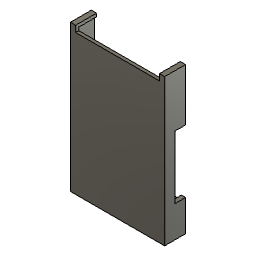
Case (Autodesk Fusion 360 archive; units mm, degrees)
design "Back Plate"
Autodesk Fusion 360 part; units mm, degrees
sketch "Sketch1" plane through (0, 0, 0) normal (0, 1, 0) x (1, 0, 0)
  line L0 (0, 0) -> (90, 0)
  line L1 (90, 0) -> (90, 20)
  line L2 (90, 20) -> (0, 20)
  line L3 (0, 20) -> (0, 0)
  dimension "d1" = 90
  dimension "d2" = 20
  constraint horizontal L0
  constraint vertical L1
  constraint horizontal L2
  constraint vertical L3
  constraint coincident L0.start L3.end
  measures "d1" distance of L0.start L0.end
  measures "d2" distance of L0.start L2.end
extrude "Extrude1" add sketch "Sketch1" along normal blind 140
shell "Shell1" thickness 3 removed faces 1 at (60, 46.6667, -20)
sketch "Sketch2" plane through (0, 0, -20) normal (0, 0, -1) x (-1, 0, 0)
  line L0 (-3, 137) -> (-3, 3)
  line L1 (-3, 3) -> (-87, 3)
  line L2 (-87, 3) -> (-87, 137)
  line L3 (-87, 137) -> (-3, 137)
  line L4 (-90, 0) -> (0, 0)
  line L5 (0, 0) -> (0, 140)
  line L6 (0, 140) -> (-90, 140)
  line L7 (-90, 140) -> (-90, 0)
  line L8 (-87, 30) -> (-90, 30)
  line L9 (-90, 30) -> (-90, 90)
  line L10 (-90, 90) -> (-87, 90)
  line L11 (-87, 90) -> (-87, 30)
  line L12 (0, 3) -> (-3, 3)
  line L13 (-3, 3) -> (-3, 18)
  line L14 (-3, 18) -> (0, 18)
  line L15 (0, 18) -> (0, 3)
  dimension "d6" = 60
  dimension "d9" = 30
  dimension "d10" = 15
  constraint horizontal L8
  constraint vertical L9
  constraint horizontal L10
  constraint vertical L11
  constraint coincident L7 L9.end
  constraint coincident L2 L8.start
  constraint horizontal L12
  constraint vertical L13
  constraint horizontal L14
  constraint vertical L15
  constraint coincident L5 L12.start
  measures "d6" distance of L8.start L10.end
  measures "d9" distance of L4 L8
  measures "d10" distance of L12.start L14.end
extrude "Extrude2" cut sketch "Sketch2" against normal blind 10 contours L2 L7 L8 L9 L10 L11
extrude "Extrude3" cut sketch "Sketch2" against normal blind 10 contours L0 L5 L12 L13 L14 L15
sketch "Sketch3" plane through (0, 0, -3) normal (0, 0, -1) x (-1, 0, 0)
  line L0 (-87, 3) -> (-3, 3)
  line L1 (-3, 3) -> (-3, 137)
  line L2 (-3, 137) -> (-87, 137)
  line L3 (-87, 137) -> (-87, 3)
  line L4 (-87, 30) -> (-80, 30)
  line L5 (-80, 30) -> (-80, 25)
  line L6 (-80, 25) -> (-87, 25)
  line L7 (-87, 25) -> (-87, 30)
  line L8 (-35, 30) -> (-28, 30)
  line L9 (-28, 30) -> (-28, 25)
  line L10 (-28, 25) -> (-35, 25)
  line L11 (-35, 25) -> (-35, 30)
  dimension "d13" = 45
  constraint horizontal L4
  constraint vertical L5
  constraint horizontal L6
  constraint vertical L7
  constraint coincident L3 L4.start
  constraint horizontal L8
  constraint vertical L9
  constraint horizontal L10
  constraint vertical L11
  measures "d13" distance of L5 L11
extrude "Extrude4" add sketch "Sketch3" along normal blind 17 contours L3 L4 L5 L6 L7 | L8 L9 L10 L11
sketch "Sketch4" plane through (0, 0, -20) normal (0, 0, -1) x (-1, 0, 0)
  line L0 (-35, 25) -> (-28, 25)
  line L1 (-28, 25) -> (-28, 30)
  line L2 (-28, 30) -> (-35, 30)
  line L3 (-35, 30) -> (-35, 25)
  line L4 (-35, 30.6629) -> (-29, 30.6629)
  line L5 (-29, 30.6629) -> (-29, 26)
  line L6 (-29, 26) -> (-35, 26)
  line L7 (-35, 26) -> (-35, 30.6629)
  constraint horizontal L4
  constraint vertical L5
  constraint horizontal L6
  constraint vertical L7
  constraint coincident L3 L4.start
sketch "Sketch5" plane through (0, 0, -20) normal (0, 0, -1) x (-1, 0, 0)
  line L0 (0, 3) -> (-87, 3)
  line L1 (-87, 3) -> (-87, 25)
  line L2 (-87, 25) -> (-80, 25)
  line L3 (-80, 25) -> (-80, 30)
  line L4 (-80, 30) -> (-90, 30)
  line L5 (-90, 30) -> (-90, 0)
  line L6 (-90, 0) -> (0, 0)
  line L7 (0, 0) -> (0, 3)
  line L8 (-80, 30) -> (-86, 30)
  line L9 (-86, 30) -> (-86, 26)
  line L10 (-86, 26) -> (-80, 26)
  line L11 (-80, 26) -> (-80, 30)
  constraint horizontal L8
  constraint vertical L9
  constraint horizontal L10
  constraint vertical L11
  constraint coincident L3.end L4.start
extrude "Extrude5" cut sketch "Sketch5" sketch "Sketch4" against normal blind 17 contours L3 L4 L8 L9 L10 L11 of sketch 2 contours L2 L4 L5 L7
extrude "Extrude6" cut sketch "Sketch4" against normal blind 17 contours L2 L3 L5 L6 L7
sketch "Sketch6" plane through (0, 0, -3) normal (0, 0, -1) x (-1, 0, 0)
  line L0 (-29, 30) -> (-28, 30)
  line L1 (-28, 30) -> (-28, 25)
  line L2 (-28, 25) -> (-35, 25)
  line L3 (-35, 25) -> (-35, 26)
  line L4 (-35, 26) -> (-29, 26)
  line L5 (-29, 26) -> (-29, 30)
  line L6 (-87, 30) -> (-86, 30)
  line L7 (-86, 30) -> (-86, 26)
  line L8 (-86, 26) -> (-80, 26)
  line L9 (-80, 26) -> (-80, 25)
  line L10 (-80, 25) -> (-87, 25)
  line L11 (-87, 25) -> (-87, 3)
  line L12 (-87, 3) -> (-3, 3)
  line L13 (-3, 3) -> (-3, 137)
  line L14 (-3, 137) -> (-87, 137)
  line L15 (-87, 137) -> (-87, 30)
  line L16 (-43, 3) -> (-48, 3)
  line L17 (-48, 3) -> (-48, 7)
  line L18 (-48, 7) -> (-43, 7)
  line L19 (-43, 7) -> (-43, 3)
  line L20 (-43, 7) -> (-47, 7)
  line L21 (-47, 7) -> (-47, 3)
  line L22 (-47, 3) -> (-43, 3)
  line L23 (-43, 3) -> (-43, 7)
  dimension "d20" = 40
  constraint horizontal L16
  constraint vertical L17
  constraint horizontal L18
  constraint vertical L19
  constraint coincident L12 L16.start
  constraint horizontal L20
  constraint vertical L21
  constraint horizontal L22
  constraint vertical L23
  constraint coincident L12 L21.end
  measures "d20" distance of L13 L19
extrude "Extrude7" add sketch "Sketch6" along normal blind 17 contours L12 L16 L17 L18 L21
sketch "Sketch7" plane through (0, 0, -3) normal (0, 0, -1) x (-1, 0, 0)
  line L0 (-48, 3) -> (-48, 7)
  line L1 (-48, 7) -> (-47, 7)
  line L2 (-47, 7) -> (-47, 3)
  line L3 (-47, 3) -> (-3, 3)
  line L4 (-3, 3) -> (-3, 137)
  line L5 (-3, 137) -> (-87, 137)
  line L6 (-87, 137) -> (-87, 30)
  line L7 (-87, 30) -> (-86, 30)
  line L8 (-86, 30) -> (-86, 26)
  line L9 (-86, 26) -> (-80, 26)
  line L10 (-80, 26) -> (-80, 25)
  line L11 (-80, 25) -> (-87, 25)
  line L12 (-87, 25) -> (-87, 3)
  line L13 (-87, 3) -> (-48, 3)
  line L14 (-29, 30) -> (-28, 30)
  line L15 (-28, 30) -> (-28, 25)
  line L16 (-28, 25) -> (-35, 25)
  line L17 (-35, 25) -> (-35, 26)
  line L18 (-35, 26) -> (-29, 26)
  line L19 (-29, 26) -> (-29, 30)
  line L20 (-47, 3) -> (-3, 3)
  line L21 (-3, 3) -> (-3, 18)
  line L22 (-3, 18) -> (-47, 18)
  line L23 (-47, 18) -> (-47, 3)
  constraint horizontal L20
  constraint vertical L21
  constraint horizontal L22
  constraint vertical L23
  constraint coincident L4 L21.end
  constraint coincident L2.end L3.start
extrude "Extrude8" add sketch "Sketch7" along normal blind 7 contours L2 L3 L4 L20 L21 L22 L23
extrude "Extrude9" add 1 faces at (47.6667, 7, -11) along direction (0, 1, 0) blind 11
sketch "Sketch8" plane through (0, 140, 0) normal (0, 1, 0) x (-1, 0, 0)
  line L0 (0, -20) -> (0, 0)
  line L1 (0, 0) -> (-90, 0)
  line L2 (-90, 0) -> (-90, -20)
  line L3 (-90, -20) -> (0, -20)
  line L4 (-90, -8) -> (-85, -8) construction
  line L5 (-85, -20) -> (-5, -20)
  line L6 (-5, -20) -> (-5, 0)
  line L7 (-5, 0) -> (-85, 0)
  line L8 (-85, 0) -> (-85, -20)
  dimension "d27" = 5
  constraint coincident L2 L4.start
  constraint perpendicular L2 L4
  constraint horizontal L5
  constraint vertical L6
  constraint horizontal L7
  constraint vertical L8
  constraint coincident L1 L6.end
  constraint coincident L3 L5.start
  measures "d27" distance of L4.start L4.end
extrude "Extrude10" cut sketch "Sketch8" against normal blind 6 contours L1 L3 L5 L6 L7 L8
